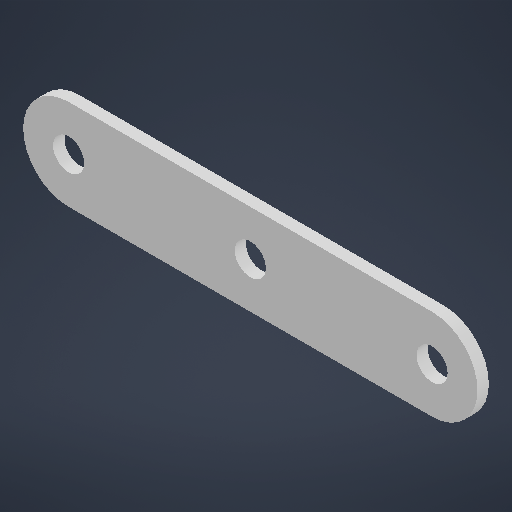
# Autodesk Inventor part: gearbox bracket
Saved by Autodesk Inventor 2025.1 (Build 291241000, 241)
## iProperties
Created: 2025-01-15
Part Number: gearbox bracket
Material: Generic
Document SubType Name: Modeling
Designer: Jahan
Density: 1 g/cm^3
Appearance: Default
Author: Jahan
Autodesk Inventor part; units mm, degrees
ref_plane "YZ Plane" through (0, 0, 0) normal (1, 0, 0) x (0, 1, 0)
ref_plane "XZ Plane" through (0, 0, 0) normal (0, 1, 0) x (-1, 0, 0)
ref_plane "XY Plane" through (0, 0, 0) normal (0, 0, 1) x (1, 0, 0)
sketch "Sketch1" plane through (0, 0, 0) normal (0, 0, 1) x (1, 0, 0)
  circle A0 centre (0, 0) radius 2.1844
  circle A1 centre (25.4, 0) radius 2.1844
  circle A2 centre (50.8, 0) radius 2.1844
  line L0 (0, 6.35) -> (50.8, 6.35)
  line L1 (0, -6.35) -> (50.8, -6.35)
  arc A3 (0, 6.35) -> (0, -6.35) centre (0, 0) ccw
  arc A4 (50.8, -6.35) -> (50.8, 6.35) centre (50.8, 0) ccw
  dimension "d0" = 4.3688
  dimension "d1" = 4.3688
  dimension "d2" = 25.4
  dimension "d3" = 4.3688
  dimension "d4" = 25.4
  constraints: 5 centre point, 4 end point, 4 point on circle, 2 tangent, 1 coincident
  measures "d0" diameter of A0
  measures "d1" diameter of A1
  measures "d2" distance of A1.centre point (0, 0)
  measures "d3" diameter of A2
  measures "d4" distance of A2.centre A1.centre
extrude "Extrusion1" add sketch "Sketch1" along normal blind 1.5875
body "Solid1"
